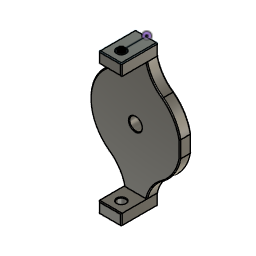
vacuum_pump_cover v3 (Autodesk Fusion 360 design; units mm, degrees)
Autodesk Fusion 360 part; units mm, degrees
note: some values were not read from the file. Set by a fixed rule: which sketch regions a step uses.
sketch "Sketch1" plane through (0, 0, 0) normal (0, 1, 0) x (1, 0, 0)
  line L0 (0, 23.75) -> (0, -23.75)
  circle A0 centre (0, 0) radius 14
  circle A1 centre (0, 0) radius 16
  line L1 (-24, 3) -> (-19.73, 6)
  line L2 (-24, 3) -> (-15.7162, 3)
  line L3 (-24, -3) -> (-24, 3)
  line L4 (-24, -3) -> (-19.73, -6)
  line L5 (-19.73, -6) -> (-9.6272, -12.7795)
  arc A2 (-4, -21) -> (-9.6272, -12.7795) centre (-17.1196, -23.9446) ccw
  line L6 (0, -21) -> (-4, -21)
  arc A3 (9.6272, -12.7795) -> (4, -21) centre (17.1196, -23.9446) ccw
  line L7 (0, -21) -> (-9.6272, -21)
  line L8 (-9.6272, -12.7795) -> (-9.6272, -23.75)
  line L9 (15.73, 23.75) -> (15.73, -38.25)
  line L10 (9.6272, -12.7795) -> (15.73, -12.7795)
  arc A4 (15.73, -21) -> (9.6272, -12.7795) centre (-22.0081, -42.6408) ccw
  line L11 (9.6272, 12.7795) -> (15.73, 12.7795)
  arc A5 (4, 21) -> (9.6272, 12.7795) centre (17.1196, 23.9446) ccw
  line L12 (4, 21) -> (-4, 21)
  arc A6 (-9.6272, 12.7795) -> (-4, 21) centre (-17.1196, 23.9446) ccw
  line L13 (7.8284, 24.4933) -> (7.8284, 23.75)
  line L14 (0, 23.75) -> (14, 23.75)
  line L15 (19.73, 23.75) -> (-19.73, 23.75)
  line L16 (-19.73, 23.75) -> (-19.73, -38.25)
  line L17 (-19.73, -38.25) -> (19.73, -38.25)
  line L18 (19.73, -38.25) -> (19.73, 23.75)
  line L19 (19.73, 23.75) -> (15.73, 23.75)
  line L20 (4, -21) -> (4, -25)
  line L21 (-4, -21) -> (-4, -25)
  line L22 (-4, -25) -> (4, -25)
  line L23 (4, 21) -> (4, 25)
  line L24 (4, 25) -> (-4, 25)
  line L25 (-4, 25) -> (-4, 21)
  line L26 (0, -21) -> (4, -21)
  circle A7 centre (0, 0) radius 2.25
  dimension "d1" = 19.73
  dimension "d2" = 14
  dimension "d3" = 28
  dimension "d4" = 32
  dimension "d5" = 6
  dimension "d6" = 4
  dimension "d8" = 47.5
  dimension "d11" = 4
  dimension "d21" = 4.5
  constraint concentric A0 A1
  constraint coincident L2.end A1
  constraint coincident L15.start L18.end
  constraint perpendicular L18 L19
  constraint coincident L9.end L17
  constraint perpendicular L9 L17
  constraint coincident L5.end A1
  constraint coincident L13.end L15
  constraint perpendicular L13 L15
  constraint coincident L7.end L8
  constraint perpendicular L7 L8
  constraint coincident A4.start L9
  constraint tangent L5 A2
  constraint coincident L10.end L9
  constraint perpendicular L9 L10
  constraint coincident L11.end L9
  constraint perpendicular L9 L11
  constraint coincident A0.centre A1.centre
  constraint perpendicular L6 L21
  constraint perpendicular L21 L22
  constraint perpendicular L15 L23
  constraint perpendicular L23 L24
  constraint perpendicular L20 L26
  measures "d1" distance of L0.start L15.start
  measures "d2" distance of L0.start L14.end
  measures "d3" diameter of A0
  measures "d4" diameter of A1
  measures "d5" distance of L1.start L3.start
  measures "d6" distance of L9.start L15.start
  measures "d8" distance of L0.start L0.end
  measures "d11" distance of A3.end L20.end
  measures "d21" diameter of A7
extrude "Extrude1" add sketch "Sketch1" against normal blind 4 contours L0 A1 A5 L12 | L0 A1 L12 A6 | L0 A0 A1 A3 L9 A5 | L0 A0 A1 A2 A6 | L0 A0 A7 | L0 A0 A7 | L0 A1 A3 L26 | L0 A1 A2 L6 L7 makes body 1
extrude "Extrude2" add sketch "Sketch1" against normal blind 13 separate body contours L0 L12 L14 L15 L23 | L14 L15 L23 L24 L25 | L0 L12 L15 L25 | L6 L7 L20 L21 L22 L26 makes body 2 at (-1.3333, -4.3333, 21) makes body 3 at (1.3333, -4.3333, -25)
sketch "Sketch2" plane through (0, 0, 25) normal (0, 0, 1) x (-1, 0, 0)
  line L0 (-4, 0) -> (4, 0)
  line L1 (4, 0) -> (4, 13)
  line L2 (4, 13) -> (-4, 13)
  line L3 (-4, 13) -> (-4, 0)
  line L4 (0, 0) -> (0, 9)
  circle A0 centre (0, 9) radius 1.475
  dimension "d14" = 9
  dimension "d15" = 2.95
  constraint coincident L4.start origin
  constraint perpendicular L0 L4
  constraint coincident L4.end A0.centre
  measures "d14" distance of L4.start L4.end
  measures "d15" diameter of A0
sketch "Sketch3" plane through (0, 0, -25) normal (0, 0, -1) x (1, 0, 0)
  line L0 (-4, 0) -> (4, 0)
  line L1 (4, 0) -> (4, 13)
  line L2 (4, 13) -> (-4, 13)
  line L3 (-4, 13) -> (-4, 0)
  line L4 (0, 0) -> (0, 9)
  circle A0 centre (0, 9) radius 1.475
  dimension "d16" = 2.95
  constraint coincident L4.start origin
  constraint perpendicular L0 L4
  constraint coincident L4.end A0.centre
  measures "d16" diameter of A0
extrude "Extrude3" cut sketch "Sketch3" against normal blind 4 contours A0 bodies 3
extrude "Extrude4" cut sketch "Sketch2" against normal blind 4 contours A0 bodies 2
fillet "Fillet1" radius 0.3 34 edges at (-16, -4, 0) (-6.0242, -4, 16.3494) (-6.0242, -4, -16.3494) (6.0242, -4, -16.3494) (13.602, -4, -8.4252) (15.73, -4, 0) (13.602, -4, 8.4252) (6.0242, -4, 16.3494) (6.0242, 0, 16.3494) (13.602, 0, 8.4252) (15.73, 0, 0) (13.602, 0, -8.4252) (6.0242, 0, -16.3494) (-6.0242, 0, -16.3494) (-16, 0, 0) (-6.0242, 0, 16.3494) (-4, -6.5, 25) (4, -6.5, 25) (0, -13, 25) (0, -13, 21) (-4, -13, 23) (4, -13, 23) (-4, 0, 23) (4, 0, 23) (0, 0, 25) (-4, -6.5, -25) (0, -13, -25) (4, -6.5, -25) (-4, -13, -23) (4, -13, -23) (0, -13, -21) (4, 0, -23) (0, 0, -25) (-4, 0, -23) on bodies 1 2 3
fillet "Fillet2" radius 0.2 5 edges at (-2.0977, -4, 0.8136) (1.3752, -9.5334, 25) (1.3752, -8.4666, 21) (-1.3752, -8.4666, -21) (-1.3752, -9.5334, -25) on bodies 1 2 3
